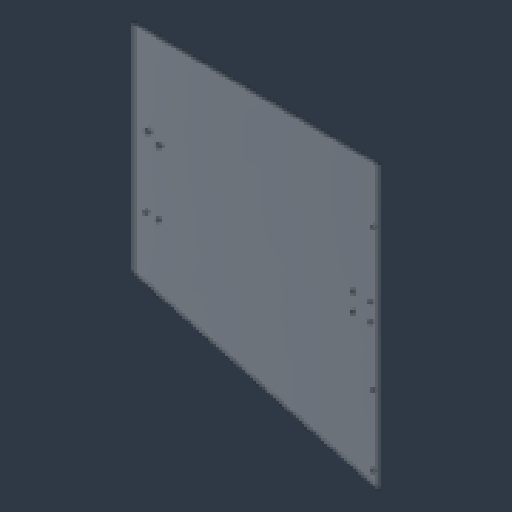
# Autodesk Inventor part: hopper_side_l
Saved by Autodesk Inventor 2024.3 (Build 283343000, 343)
## iProperties
Created: 2025-03-07
Part Number: hopper_side_l
Material: Polycarbonate, Clear
Document SubType Name: Sheet Metal
Designer: marcu
Density: 1.2 g/cm^3
Sheet Metal Rule: Default
Appearance: Polycarbonate - Clear
Author: marcu
Autodesk Inventor part; units mm, degrees
ref_plane "YZ Plane" through (0, 0, 0) normal (1, 0, 0) x (0, 1, 0)
ref_plane "XZ Plane" through (0, 0, 0) normal (0, 1, 0) x (-1, 0, 0)
ref_plane "XY Plane" through (0, 0, 0) normal (0, 0, 1) x (1, 0, 0)
sketch "Sketch1" plane through (0, 0, 0) normal (0, 0, 1) x (1, 0, 0)
  line L0 (-177.8, 203.2) -> (177.8, 203.2)
  line L1 (177.8, 203.2) -> (177.8, -203.2)
  line L2 (177.8, -203.2) -> (-177.8, -203.2)
  line L3 (-177.8, -203.2) -> (-177.8, 203.2)
  line L4 (-177.8, 203.2) -> (177.8, -203.2) construction
  line L5 (177.8, 203.2) -> (-177.8, -203.2) construction
  point P0 (0, 0)
  dimension "d0" = 355.6
  dimension "d1" = 406.4
  measures "d0" distance of L1.end L2.end
  measures "d1" distance of L0.end L1.end
extrude "Plate1" add sketch "Sketch1" along normal blind 3.048
sketch "Sketch2" plane through (0, 0, 0) normal (0, 0, -1) x (-1, 0, 0)
  line L0 (177.8, -203.2) -> (-177.8, -203.2) construction
  line L1 (177.8, 203.2) -> (177.8, -203.2) construction
  line L2 (-177.8, 203.2) -> (177.8, 203.2) construction
  line L3 (-177.8, -203.2) -> (-177.8, 203.2) construction
  line L4 (-177.8, -203.2) -> (177.8, -107.9173)
  line L5 (-177.8, -203.2) -> (190.3442, -203.2) construction
  line L6 (177.8, 203.2) -> (177.8, -203.2) construction
  line L7 (177.8, -107.9173) -> (177.8, -203.2)
  line L8 (177.8, -203.2) -> (-177.8, -203.2)
  point P0 (0, 0)
  dimension "d3" = 15
  constraints: 8 end point, 2 collinear, 2 point on line, 1 equal length, 1 horizontal
  measures "d3" angle of L5 L4
extrude "Cut1" cut sketch "Sketch2" against normal blind 3.048
sketch "Sketch3" plane through (0, 0, 0) normal (0, 0, -1) x (-1, 0, 0)
  line L0 (-177.8, -203.2) -> (177.8, -107.9173) construction
  line L1 (177.8, 203.2) -> (177.8, -107.9173) construction
  line L2 (-177.8, 203.2) -> (177.8, 203.2) construction
  line L3 (-177.8, -203.2) -> (-177.8, 203.2) construction
  line L4 (-177.8, 0) -> (-165.1, 0) construction
  point P0 (0, 0)
  point P1 (-139.7, 0)
  point P2 (-165.1, 25.4)
  point P3 (-139.7, 25.4)
  dimension "d6" = 12.7
  dimension "d9" = 25.4
  dimension "d12" = 25.4
  constraints: 2 end point, 2 horizontal, 1 coincident, 1 midpoint, 1 vertical, 3 other
  measures "d6" distance of L4.start L4.end
  measures "d9" distance of point (-165.1, 0) point (-139.7, 0)
  measures "d12" distance of point (-165.1, 0) point (-165.1, 25.4)
hole "Hole1" at (165.1, 0, 0) at (139.7, 0, 0) at (165.1, 25.4, 0) at (139.7, 25.4, 0) direction (0, 0, 1) diameter 5.1054 end through all clearance for "Flat Head Machine Screw (82)" size "#10" standard "Ansi Unified Screw Threads"
sketch "Sketch4" plane through (0, 0, 0) normal (0, 0, -1) x (-1, 0, 0)
  line L0 (-168.8973, -203.2) -> (-168.8973, 203.2) construction
  line L1 (-177.8, -203.2) -> (-177.8, 203.2) projected
  point P0 (0, 0)
  point P1 (-168.8973, -184.15)
  point P2 (-168.8973, -82.55)
  point P3 (-168.8973, 120.65)
  dimension "d22" = 8.9027
  dimension "d23" = 101.6
  dimension "d24" = 19.05
  dimension "d25" = 203.2
  constraints: 3 point on line, 2 end point, 2 horizontal alignment, 1 parallel
  measures "d22" distance between parallel lines of L1 L0
  measures "d23" distance of point (-168.897, -82.55) point (-168.897, -184.15)
  measures "d24" distance of L0.start point (-168.897, -184.15)
  measures "d25" distance of point (-168.897, -82.55) point (-168.897, 120.65)
hole "Hole2" at (168.8973, -184.15, 0) at (168.8973, -82.55, 0) at (168.8973, 120.65, 0) direction (0, 0, 1) diameter 5.1054 end through all
sketch "Sketch5" plane through (0, 0, 0) normal (0, 0, -1) x (-1, 0, 0)
  circle A0 centre (158.75, -25.1401) radius 2.0193 projected
  circle A1 centre (139.7074, -24.6077) radius 2.0193 projected
  point P0 (0, 0)
hole "Hole3" at (-158.75, -25.1401, 0) at (-139.7074, -24.6077, 0) direction (0, 0, 1) diameter 5.1054 depth 3.048 tip angle 118
sketch "Sketch6" plane through (0, 0, 3.048) normal (0, 0, 1) x (1, 0, 0)
  line L0 (-155.0242, 77.8222) -> (-152.7105, 76.4193)
  line L1 (-177.8, -107.9173) -> (-177.8, 203.2) projected
  point P0 (0, 0)
  point P1 (-155.575, 78.1562)
  point P2 (-139.2858, 68.2788)
  dimension "d40" = 19.05
  dimension "d41" = 22.225
  constraints: 2 end point, 2 point on line, 3 other
  measures "d40" distance of point (-155.575, 78.156) point (-139.286, 68.279)
  measures "d41" distance from line of L1 point (-155.575, 78.156)
hole "Hole4" at (-155.575, 78.1562, 3.048) at (-139.2858, 68.2788, 3.048) direction (0, 0, -1) diameter 6.35 depth 3.048 tip angle 118
equation "\"d4\" = Thickness"
equation "\"d20\" = Thickness"
equation "\"d31\" = Thickness"
equation "\"d38\" = Thickness"
equation "\"d47\" = Thickness"
equation "\"d2\" = Thickness"
equation "\"BendRadius\" = Thickness"
equation "\"BendReliefWidth\" = Thickness"
equation "\"BendReliefDepth\" = 0.5 * Thickness"
equation "\"CornerReliefSize\" = 4 * Thickness"
equation "\"MinimumRemnant\" = 2 * Thickness"
equation "\"TransitionRadius\" = BendRadius"
equation "\"JacobiRadiusSize\" = BendRadius"
equation "\"GapSize\" = Thickness"
equation "\"Thickness\" = 3.048"
body "Solid1"
